Autodesk Fusion 360 part; units mm, degrees
(part 2 of 2)
sketch "Sketch37" plane through (0, 34, 0) normal (0, -1, 0) x (1, 0, 0)
  line L0 (112, 0) -> (98, 0)
  line L1 (98, 0) -> (98, -4.6)
  line L2 (98, -4.6) -> (112, -4.6)
  line L3 (112, -4.6) -> (112, 0)
  line L4 (105, 0) -> (105, -2.1)
  line L5 (107, -2.8) -> (103, -2.8)
  line L6 (103, -2.8) -> (103, -1.4)
  line L7 (103, -1.4) -> (107, -1.4)
  line L8 (107, -1.4) -> (107, -2.8)
  line L9 (107, -2.8) -> (103, -1.4) construction
  line L10 (103, -2.8) -> (107, -1.4) construction
  point P0 (105, -2.1)
  dimension "d205" = 2.1
  dimension "d206" = 4
  dimension "d207" = 1.4
  constraint midpoint L0 L4.start
  constraint perpendicular L0 L4
  constraint horizontal L5
  constraint perpendicular L5 L6
  constraint parallel L5 L7
  constraint parallel L6 L8
  constraint coincident L9 P0
  constraint coincident L10 P0
  constraint coincident P0 L4.end
  measures "d205" distance of L4.start P0
  measures "d206" distance of L6.end L7.end
  measures "d207" distance of L5.end L6.end
extrude "Extrude38" cut sketch "Sketch37" against normal blind 1 contours L5 L6 L7 L8
sketch "Sketch38" plane through (0, 50, 0) normal (0, -1, 0) x (1, 0, 0)
  line L0 (141, 0) -> (127, 0)
  line L1 (127, 0) -> (127, -4.6)
  line L2 (127, -4.6) -> (141, -4.6)
  line L3 (141, -4.6) -> (141, 0)
  line L4 (134, 0) -> (134, -2.1)
  line L5 (136, -2.8) -> (132, -2.8)
  line L6 (132, -2.8) -> (132, -1.4)
  line L7 (132, -1.4) -> (136, -1.4)
  line L8 (136, -1.4) -> (136, -2.8)
  line L9 (136, -2.8) -> (132, -1.4) construction
  line L10 (132, -2.8) -> (136, -1.4) construction
  point P0 (134, -2.1)
  dimension "d210" = 2.1
  dimension "d211" = 4
  dimension "d212" = 1.4
  constraint midpoint L0 L4.start
  constraint perpendicular L0 L4
  constraint horizontal L5
  constraint perpendicular L5 L6
  constraint parallel L5 L7
  constraint parallel L6 L8
  constraint coincident L9 P0
  constraint coincident L10 P0
  constraint coincident P0 L4.end
  measures "d210" distance of L4.start P0
  measures "d211" distance of L6.end L7.end
  measures "d212" distance of L5.end L6.end
extrude "Extrude39" cut sketch "Sketch38" against normal blind 1 contours L5 L6 L7 L8
sketch "Sketch39" plane through (0, 36, 0) normal (0, 1, 0) x (-1, 0, 0)
  line L0 (-127, 0) -> (-141, 0)
  line L1 (-141, 0) -> (-141, -4.6)
  line L2 (-141, -4.6) -> (-127, -4.6)
  line L3 (-127, -4.6) -> (-127, 0)
  line L4 (-134, 0) -> (-134, -2.1)
  line L5 (-132, -2.8) -> (-136, -2.8)
  line L6 (-136, -2.8) -> (-136, -1.4)
  line L7 (-136, -1.4) -> (-132, -1.4)
  line L8 (-132, -1.4) -> (-132, -2.8)
  line L9 (-132, -2.8) -> (-136, -1.4) construction
  line L10 (-136, -2.8) -> (-132, -1.4) construction
  point P0 (-134, -2.1)
  dimension "d215" = 2.1
  dimension "d216" = 4
  dimension "d217" = 1.4
  constraint midpoint L0 L4.start
  constraint perpendicular L0 L4
  constraint horizontal L5
  constraint perpendicular L5 L6
  constraint parallel L5 L7
  constraint parallel L6 L8
  constraint coincident L9 P0
  constraint coincident L10 P0
  constraint coincident P0 L4.end
  measures "d215" distance of L4.start P0
  measures "d216" distance of L6.end L7.end
  measures "d217" distance of L5.end L6.end
extrude "Extrude40" cut sketch "Sketch39" against normal blind 1 contours L5 L6 L7 L8
sketch "Sketch40" plane through (0, 17, 0) normal (0, 1, 0) x (-1, 0, 0)
  line L0 (-127, 0) -> (-141, 0)
  line L1 (-141, 0) -> (-141, -4.6)
  line L2 (-141, -4.6) -> (-127, -4.6)
  line L3 (-127, -4.6) -> (-127, 0)
  line L4 (-134, 0) -> (-134, -2.1)
  line L5 (-132, -2.8) -> (-136, -2.8)
  line L6 (-136, -2.8) -> (-136, -1.4)
  line L7 (-136, -1.4) -> (-132, -1.4)
  line L8 (-132, -1.4) -> (-132, -2.8)
  line L9 (-132, -2.8) -> (-136, -1.4) construction
  line L10 (-136, -2.8) -> (-132, -1.4) construction
  point P0 (-134, -2.1)
  dimension "d220" = 2.1
  dimension "d221" = 4
  dimension "d222" = 1.4
  constraint midpoint L0 L4.start
  constraint perpendicular L0 L4
  constraint horizontal L5
  constraint perpendicular L5 L6
  constraint parallel L5 L7
  constraint parallel L6 L8
  constraint coincident L9 P0
  constraint coincident L10 P0
  constraint coincident P0 L4.end
  measures "d220" distance of L4.start P0
  measures "d221" distance of L6.end L7.end
  measures "d222" distance of L5.end L6.end
extrude "Extrude41" cut sketch "Sketch40" against normal blind 1 contours L5 L6 L7 L8
sketch "Sketch41" plane through (0, 31, 0) normal (0, -1, 0) x (1, 0, 0)
  line L0 (141, 0) -> (127, 0)
  line L1 (127, 0) -> (127, -4.6)
  line L2 (127, -4.6) -> (141, -4.6)
  line L3 (141, -4.6) -> (141, 0)
  line L4 (134, 0) -> (134, -2.1)
  line L5 (136, -2.8) -> (132, -2.8)
  line L6 (132, -2.8) -> (132, -1.4)
  line L7 (132, -1.4) -> (136, -1.4)
  line L8 (136, -1.4) -> (136, -2.8)
  line L9 (136, -2.8) -> (132, -1.4) construction
  line L10 (132, -2.8) -> (136, -1.4) construction
  point P0 (134, -2.1)
  dimension "d225" = 2.1
  dimension "d226" = 4
  dimension "d227" = 1.4
  constraint midpoint L0 L4.start
  constraint perpendicular L0 L4
  constraint horizontal L5
  constraint perpendicular L5 L6
  constraint parallel L5 L7
  constraint parallel L6 L8
  constraint coincident L9 P0
  constraint coincident L10 P0
  constraint coincident P0 L4.end
  measures "d225" distance of L4.start P0
  measures "d226" distance of L6.end L7.end
  measures "d227" distance of L5.end L6.end
extrude "Extrude42" cut sketch "Sketch41" against normal blind 1 contours L5 L6 L7 L8
sketch "Sketch42" plane through (0, 34, 0) normal (0, -1, 0) x (1, 0, 0)
  line L0 (167, 0) -> (153, 0)
  line L1 (153, 0) -> (153, -4.6)
  line L2 (153, -4.6) -> (167, -4.6)
  line L3 (167, -4.6) -> (167, 0)
  line L4 (160, 0) -> (160, -2.1)
  line L5 (162, -2.8) -> (158, -2.8)
  line L6 (158, -2.8) -> (158, -1.4)
  line L7 (158, -1.4) -> (162, -1.4)
  line L8 (162, -1.4) -> (162, -2.8)
  line L9 (162, -2.8) -> (158, -1.4) construction
  line L10 (158, -2.8) -> (162, -1.4) construction
  point P0 (160, -2.1)
  dimension "d230" = 2.1
  dimension "d231" = 4
  dimension "d232" = 1.4
  constraint midpoint L0 L4.start
  constraint perpendicular L0 L4
  constraint horizontal L5
  constraint perpendicular L5 L6
  constraint parallel L5 L7
  constraint parallel L6 L8
  constraint coincident L9 P0
  constraint coincident L10 P0
  constraint coincident P0 L4.end
  measures "d230" distance of L4.start P0
  measures "d231" distance of L6.end L7.end
  measures "d232" distance of L5.end L6.end
extrude "Extrude43" cut sketch "Sketch42" against normal blind 1 contours L5 L6 L7 L8
sketch "Sketch43" plane through (0, 20, 0) normal (0, 1, 0) x (-1, 0, 0)
  line L0 (-153, 0) -> (-167, 0)
  line L1 (-167, 0) -> (-167, -4.6)
  line L2 (-167, -4.6) -> (-153, -4.6)
  line L3 (-153, -4.6) -> (-153, 0)
  line L4 (-160, 0) -> (-160, -2.1)
  line L5 (-158, -2.8) -> (-162, -2.8)
  line L6 (-162, -2.8) -> (-162, -1.4)
  line L7 (-162, -1.4) -> (-158, -1.4)
  line L8 (-158, -1.4) -> (-158, -2.8)
  line L9 (-158, -2.8) -> (-162, -1.4) construction
  line L10 (-162, -2.8) -> (-158, -1.4) construction
  point P0 (-160, -2.1)
  dimension "d235" = 2.1
  dimension "d236" = 4
  dimension "d237" = 1.4
  constraint midpoint L0 L4.start
  constraint perpendicular L0 L4
  constraint horizontal L5
  constraint perpendicular L5 L6
  constraint parallel L5 L7
  constraint parallel L6 L8
  constraint coincident L9 P0
  constraint coincident L10 P0
  constraint coincident P0 L4.end
  measures "d235" distance of L4.start P0
  measures "d236" distance of L6.end L7.end
  measures "d237" distance of L5.end L6.end
extrude "Extrude44" cut sketch "Sketch43" against normal blind 1 contours L5 L6 L7 L8
sketch "Sketch44" plane through (0, 1, 0) normal (0, 1, 0) x (-1, 0, 0)
  line L0 (-153, 0) -> (-167, 0)
  line L1 (-167, 0) -> (-167, -4.6)
  line L2 (-167, -4.6) -> (-153, -4.6)
  line L3 (-153, -4.6) -> (-153, 0)
  line L4 (-160, 0) -> (-160, -2.1)
  line L5 (-158, -2.8) -> (-162, -2.8)
  line L6 (-162, -2.8) -> (-162, -1.4)
  line L7 (-162, -1.4) -> (-158, -1.4)
  line L8 (-158, -1.4) -> (-158, -2.8)
  line L9 (-158, -2.8) -> (-162, -1.4) construction
  line L10 (-162, -2.8) -> (-158, -1.4) construction
  point P0 (-160, -2.1)
  dimension "d240" = 2.1
  dimension "d241" = 4
  dimension "d242" = 1.4
  constraint midpoint L0 L4.start
  constraint perpendicular L0 L4
  constraint horizontal L5
  constraint perpendicular L5 L6
  constraint parallel L5 L7
  constraint parallel L6 L8
  constraint coincident L9 P0
  constraint coincident L10 P0
  constraint coincident P0 L4.end
  measures "d240" distance of L4.start P0
  measures "d241" distance of L6.end L7.end
  measures "d242" distance of L5.end L6.end
extrude "Extrude45" cut sketch "Sketch44" against normal blind 1 contours L5 L6 L7 L8
sketch "Sketch45" plane through (0, 15, 0) normal (0, -1, 0) x (1, 0, 0)
  line L0 (167, 0) -> (153, 0)
  line L1 (153, 0) -> (153, -4.6)
  line L2 (153, -4.6) -> (167, -4.6)
  line L3 (167, -4.6) -> (167, 0)
  line L4 (160, 0) -> (160, -2.1)
  line L5 (162, -2.8) -> (158, -2.8)
  line L6 (158, -2.8) -> (158, -1.4)
  line L7 (158, -1.4) -> (162, -1.4)
  line L8 (162, -1.4) -> (162, -2.8)
  line L9 (162, -2.8) -> (158, -1.4) construction
  line L10 (158, -2.8) -> (162, -1.4) construction
  point P0 (160, -2.1)
  dimension "d245" = 2.1
  dimension "d246" = 4
  dimension "d247" = 1.4
  constraint midpoint L0 L4.start
  constraint perpendicular L0 L4
  constraint horizontal L5
  constraint perpendicular L5 L6
  constraint parallel L5 L7
  constraint parallel L6 L8
  constraint coincident L9 P0
  constraint coincident L10 P0
  constraint coincident P0 L4.end
  measures "d245" distance of L4.start P0
  measures "d246" distance of L6.end L7.end
  measures "d247" distance of L5.end L6.end
extrude "Extrude46" cut sketch "Sketch45" against normal blind 1 contours L5 L6 L7 L8
fillet "Fillet1" radius 1 8 edges at (-180.364, -66.364, 0) (-183, 0, 0) (-180.364, 66.364, 0) (0, 69, 0) (180.364, 66.364, 0) (183, 0, 0) (180.364, -66.364, 0) (0, -69, 0)
chamfer "Chamfer1" distance 0.4 angle 45 7 edges at (-170.5759, 58.0598, 0) (-170.5759, -59.9402, 0) (2.4241, -59.9402, 0) (-55.4241, 59.9402, 0) (50.5759, 59.9402, 0) (175.4241, -59.9402, 0) (175.4241, 58.0598, 0)
sketch "Sketch46" plane through (0, 0, 0) normal (0, 0, 1) x (-1, 0, 0)
  circle A0 centre (-173, 59) radius 3
  circle A1 centre (53, -59) radius 3
  circle A2 centre (173, 59) radius 3
  arc A3 (182, 60) -> (174, 68) centre (174, 60) ccw
  line L0 (174, 68) -> (-174, 68)
  arc A4 (-174, 68) -> (-182, 60) centre (-174, 60) ccw
  line L1 (-182, 60) -> (-182, -60)
  arc A5 (-182, -60) -> (-174, -68) centre (-174, -60) ccw
  line L2 (-174, -68) -> (174, -68)
  arc A6 (174, -68) -> (182, -60) centre (174, -60) ccw
  line L3 (182, -60) -> (182, 60)
  circle A7 centre (-33, -54) radius 3.5
  circle A8 centre (-33, -20) radius 3.5
  circle A9 centre (33, -54) radius 3.5
  circle A10 centre (33, -20) radius 3.5
  line L4 (60, 53) -> (60, 39)
  line L5 (60, 39) -> (46, 39)
  line L6 (46, 39) -> (46, 53)
  line L7 (46, 53) -> (60, 53)
  line L8 (-72, -27) -> (-72, -41)
  line L9 (-72, -41) -> (-86, -41)
  line L10 (-86, -41) -> (-86, -27)
  line L11 (-86, -27) -> (-72, -27)
  line L12 (-79, 0) -> (-79, 14)
  line L13 (-79, 14) -> (-65, 14)
  line L14 (-65, 14) -> (-65, 0)
  line L15 (-65, 0) -> (-79, 0)
  line L16 (-72, -22) -> (-86, -22)
  line L17 (-86, -22) -> (-86, -8)
  line L18 (-86, -8) -> (-72, -8)
  line L19 (-72, -8) -> (-72, -22)
  line L20 (141, -50) -> (127, -50)
  line L21 (127, -50) -> (127, -36)
  line L22 (127, -36) -> (141, -36)
  line L23 (141, -36) -> (141, -50)
  line L24 (-84, 13) -> (-98, 13)
  line L25 (-98, 13) -> (-98, 27)
  line L26 (-98, 27) -> (-84, 27)
  line L27 (-84, 27) -> (-84, 13)
  line L28 (72, -27) -> (86, -27)
  line L29 (86, -27) -> (86, -41)
  line L30 (86, -41) -> (72, -41)
  line L31 (72, -41) -> (72, -27)
  line L32 (112, -53) -> (98, -53)
  line L33 (98, -53) -> (98, -39)
  line L34 (98, -39) -> (112, -39)
  line L35 (112, -39) -> (112, -53)
  line L36 (-98, -39) -> (-98, -53)
  line L37 (-98, -53) -> (-112, -53)
  line L38 (-112, -53) -> (-112, -39)
  line L39 (-112, -39) -> (-98, -39)
  line L40 (-60, 13) -> (-60, 27)
  line L41 (-60, 27) -> (-46, 27)
  line L42 (-46, 27) -> (-46, 13)
  line L43 (-46, 13) -> (-60, 13)
  line L44 (79, 40) -> (79, 26)
  line L45 (79, 26) -> (65, 26)
  line L46 (65, 26) -> (65, 40)
  line L47 (65, 40) -> (79, 40)
  line L48 (167, -34) -> (153, -34)
  line L49 (153, -34) -> (153, -20)
  line L50 (153, -20) -> (167, -20)
  line L51 (167, -20) -> (167, -34)
  line L52 (-98, -20) -> (-98, -34)
  line L53 (-98, -34) -> (-112, -34)
  line L54 (-112, -34) -> (-112, -20)
  line L55 (-112, -20) -> (-98, -20)
  line L56 (-127, -50) -> (-141, -50)
  line L57 (-141, -50) -> (-141, -36)
  line L58 (-141, -36) -> (-127, -36)
  line L59 (-127, -36) -> (-127, -50)
  line L60 (-79, 40) -> (-65, 40)
  line L61 (-65, 40) -> (-65, 26)
  line L62 (-65, 26) -> (-79, 26)
  line L63 (-79, 26) -> (-79, 40)
  line L64 (-46, 53) -> (-46, 39)
  line L65 (-46, 39) -> (-60, 39)
  line L66 (-60, 39) -> (-60, 53)
  line L67 (-60, 53) -> (-46, 53)
  line L68 (7, 13) -> (-7, 13)
  line L69 (-7, 13) -> (-7, 27)
  line L70 (-7, 27) -> (7, 27)
  line L71 (7, 27) -> (7, 13)
  line L72 (-141, -31) -> (-141, -17)
  line L73 (-141, -17) -> (-127, -17)
  line L74 (-127, -17) -> (-127, -31)
  line L75 (-127, -31) -> (-141, -31)
  line L76 (-167, -1) -> (-153, -1)
  line L77 (-153, -1) -> (-153, -15)
  line L78 (-153, -15) -> (-167, -15)
  line L79 (-167, -15) -> (-167, -1)
  line L80 (-167, -20) -> (-153, -20)
  line L81 (-153, -20) -> (-153, -34)
  line L82 (-153, -34) -> (-167, -34)
  line L83 (-167, -34) -> (-167, -20)
  circle A11 centre (173, -59) radius 3
  circle A12 centre (0, 59) radius 3
  circle A13 centre (-53, -59) radius 3
  circle A14 centre (-173, -59) radius 3
  line L84 (12, 27) -> (26, 27)
  line L85 (26, 27) -> (26, 13)
  line L86 (26, 13) -> (12, 13)
  line L87 (12, 13) -> (12, 27)
  line L88 (-12, 27) -> (-26, 27)
  line L89 (-26, 27) -> (-26, 13)
  line L90 (-26, 13) -> (-12, 13)
  line L91 (-12, 13) -> (-12, 27)
  dimension "d268" = 14
  dimension "d269" = 14
  dimension "d270" = 14
  dimension "d271" = 14
  constraint horizontal L84
  constraint vertical L85
  constraint horizontal L86
  constraint vertical L87
  constraint horizontal L88
  constraint vertical L89
  constraint horizontal L90
  constraint vertical L91
  measures "d268" distance of L84.start L84.end
  measures "d269" distance of L84.start L86.end
  measures "d270" distance of L88.start L88.end
  measures "d271" distance of L88.start L90.end
extrude "Extrude48" cut sketch "Sketch46" against normal blind 4.6 contours L84 L85 L86 L87 | L88 L89 L90 L91
sketch "Sketch48" plane through (0, -27, 0) normal (0, 1, 0) x (-1, 0, 0)
  line L0 (26, 0) -> (12, 0)
  line L1 (12, 0) -> (12, -4.6)
  line L2 (12, -4.6) -> (26, -4.6)
  line L3 (26, -4.6) -> (26, 0)
  line L4 (19, 0) -> (19, -2.1)
  line L5 (21, -2.8) -> (17, -2.8)
  line L6 (17, -2.8) -> (17, -1.4)
  line L7 (17, -1.4) -> (21, -1.4)
  line L8 (21, -1.4) -> (21, -2.8)
  line L9 (21, -2.8) -> (17, -1.4) construction
  line L10 (17, -2.8) -> (21, -1.4) construction
  line L11 (-19, 0) -> (-19, -2.1)
  line L12 (-17, -2.8) -> (-21, -2.8)
  line L13 (-21, -2.8) -> (-21, -1.4)
  line L14 (-21, -1.4) -> (-17, -1.4)
  line L15 (-17, -1.4) -> (-17, -2.8)
  line L16 (-17, -2.8) -> (-21, -1.4) construction
  line L17 (-21, -2.8) -> (-17, -1.4) construction
  point P0 (19, -2.1)
  point P1 (-19, -2.1)
  dimension "d274" = 2.1
  dimension "d275" = 4
  dimension "d276" = 1.4
  dimension "d277" = 2.1
  dimension "d278" = 4
  dimension "d279" = 1.4
  constraint midpoint L0 L4.start
  constraint perpendicular L0 L4
  constraint horizontal L5
  constraint perpendicular L5 L6
  constraint parallel L5 L7
  constraint parallel L6 L8
  constraint coincident L9 P0
  constraint coincident L10 P0
  constraint coincident P0 L4.end
  constraint horizontal L12
  constraint perpendicular L12 L13
  constraint parallel L12 L14
  constraint parallel L13 L15
  constraint coincident L16 P1
  constraint coincident L17 P1
  constraint coincident P1 L11.end
  measures "d274" distance of L4.start P0
  measures "d275" distance of L6.end L7.end
  measures "d276" distance of L5.end L6.end
  measures "d277" distance of L11.start P1
  measures "d278" distance of L13.end L14.end
  measures "d279" distance of L12.end L13.end
sketch "Sketch49" plane through (0, -13, 0) normal (0, -1, 0) x (1, 0, 0)
  line L0 (-12, 0) -> (-26, 0)
  line L1 (-26, 0) -> (-26, -4.6)
  line L2 (-26, -4.6) -> (-12, -4.6)
  line L3 (-12, -4.6) -> (-12, 0)
  line L4 (-19, 0) -> (-19, -2.1)
  line L5 (-17, -2.8) -> (-21, -2.8)
  line L6 (-21, -2.8) -> (-21, -1.4)
  line L7 (-21, -1.4) -> (-17, -1.4)
  line L8 (-17, -1.4) -> (-17, -2.8)
  line L9 (-17, -2.8) -> (-21, -1.4) construction
  line L10 (-21, -2.8) -> (-17, -1.4) construction
  line L11 (19, 0) -> (19, -2.1)
  line L12 (21, -2.8) -> (17, -2.8)
  line L13 (17, -2.8) -> (17, -1.4)
  line L14 (17, -1.4) -> (21, -1.4)
  line L15 (21, -1.4) -> (21, -2.8)
  line L16 (21, -2.8) -> (17, -1.4) construction
  line L17 (17, -2.8) -> (21, -1.4) construction
  point P0 (-19, -2.1)
  point P1 (19, -2.1)
  dimension "d280" = 2.1
  dimension "d281" = 4
  dimension "d282" = 1.4
  dimension "d283" = 2.1
  dimension "d284" = 4
  dimension "d285" = 1.4
  constraint midpoint L0 L4.start
  constraint perpendicular L0 L4
  constraint horizontal L5
  constraint perpendicular L5 L6
  constraint parallel L5 L7
  constraint parallel L6 L8
  constraint coincident L9 P0
  constraint coincident L10 P0
  constraint coincident P0 L4.end
  constraint vertical L11
  constraint horizontal L12
  constraint perpendicular L12 L13
  constraint parallel L12 L14
  constraint parallel L13 L15
  constraint coincident L16 P1
  constraint coincident L17 P1
  constraint coincident P1 L11.end
  measures "d280" distance of L4.start P0
  measures "d281" distance of L6.end L7.end
  measures "d282" distance of L5.end L6.end
  measures "d283" distance of L11.start P1
  measures "d284" distance of L13.end L14.end
  measures "d285" distance of L12.end L13.end
extrude "Extrude49" cut sketch "Sketch49" against normal blind 1 contours L5 L6 L7 L8 | L12 L13 L14 L15
extrude "Extrude50" cut sketch "Sketch48" against normal blind 1 contours L5 L6 L7 L8 | L12 L13 L14 L15
